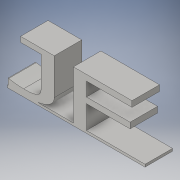
# Autodesk Inventor part: jf_inits
Saved by Autodesk Inventor 2016 (Build 200138000, 138)
## iProperties
Created: 2016-01-28
Part Number: jf_inits
Material: Generic
Document SubType Name: Modeling
Designer: jforce
Density: 1 g/cm^3
Appearance: Default
Author: jforce
Autodesk Inventor part; units mm, degrees
ref_plane "YZ Plane" through (0, 0, 0) normal (1, 0, 0) x (0, 1, 0)
ref_plane "XZ Plane" through (0, 0, 0) normal (0, 1, 0) x (-1, 0, 0)
ref_plane "XY Plane" through (0, 0, 0) normal (0, 0, 1) x (1, 0, 0)
sketch "Sketch1" plane through (0, 0, 0) normal (0, 0, 1) x (1, 0, 0)
  line L0 (0, 0) -> (50, 0) construction
  line L1 (50, 0) -> (50, 20) construction
  line L2 (50, 0.7657) -> (0, 0.7657) construction
  line L3 (0, 20) -> (0, 0) construction
  spline S0 degree 2 poles (17.0019, 5.3908) (17.0019, 3.0567) (11.2962, 0.5208) (6.4982, 0.5208) knots 0 0 0 1 2 2 2
  spline S1 degree 2 poles (6.4982, 0.5208) (5.3455, 0.5208) (1.4985, 0.7225) (0.2161, 0.8666) knots 0 0 0 1 2 2 2
  line L4 (0.2161, 0.8666) -> (0.2161, 3.1431)
  line L5 (0.2161, 3.1431) -> (0.4755, 3.1431)
  spline S2 degree 2 poles (0.4755, 3.1431) (1.4553, 2.9702) (4.3513, 2.5668) (5.8498, 2.5668) knots 0 0 0 1 2 2 2
  spline S3 degree 2 poles (5.8498, 2.5668) (8.0543, 2.5668) (10.6478, 3.0711) (11.2674, 3.5321) knots 0 0 0 1 2 2 2
  spline S4 degree 2 poles (11.2674, 3.5321) (11.9158, 4.0076) (12.276, 5.3908) (12.276, 6.2986) knots 0 0 0 1 2 2 2
  line L6 (12.276, 6.2986) -> (12.276, 16.6582)
  line L7 (12.276, 16.6582) -> (4.7548, 16.6582)
  line L8 (4.7548, 16.6582) -> (4.7548, 18.5457)
  line L9 (4.7548, 18.5457) -> (17.0019, 18.5457)
  line L10 (17.0019, 18.5457) -> (17.0019, 5.3908)
  line L11 (45.2569, 16.4421) -> (28.7016, 16.4421)
  line L12 (28.7016, 16.4421) -> (28.7016, 11.428)
  line L13 (28.7016, 11.428) -> (44.5653, 11.428)
  line L14 (44.5653, 11.428) -> (44.5653, 9.3243)
  line L15 (44.5653, 9.3243) -> (28.7016, 9.3243)
  line L16 (28.7016, 9.3243) -> (28.7016, 0.7657)
  line L17 (28.7016, 0.7657) -> (23.9756, 0.7657)
  line L18 (23.9756, 0.7657) -> (23.9756, 18.5457)
  line L19 (23.9756, 18.5457) -> (45.2569, 18.5457)
  line L20 (45.2569, 18.5457) -> (45.2569, 16.4421)
  dimension "d0" = 50
  dimension "d1" = 20
  constraints: 8 end point, 2 horizontal, 2 parallel, 1 perpendicular
  measures "d0" distance of L2.end L2.start
  measures "d1" distance of L1.end L0.end
extrude "Extrusion1" add sketch "Sketch1" along normal blind 10
sketch "Sketch2" plane through (0, 0, 0) normal (1, 0, 0) x (0, 1, 0)
  point P0 (0, 0)
sketch "Sketch3" plane through (0, 0, 0) normal (0, 0, 1) x (1, 0, 0)
  line L0 (0, 0) -> (50, 0)
  line L1 (50, 0) -> (50, 0.8967)
  line L2 (50, 0.8967) -> (0, 0.8967)
  line L3 (0, 0.8967) -> (0, 0)
  dimension "d4" = 50
  constraints: 8 end point, 2 parallel, 1 horizontal, 1 perpendicular
  measures "d4" distance of L2.end L1.end
extrude "Extrusion2" add sketch "Sketch3" along normal blind 10
body "Solid1"
